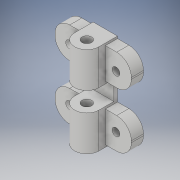
# Autodesk Inventor part: Nose Gear Mounting Block
Saved by Autodesk Inventor 2018 (Build 220112000, 112)
## iProperties
Created: 2018-08-04
Part Number: Nose Gear Mounting Block
Material: Generic
Document SubType Name: Modeling
Designer: Michael Gunderman
Density: 0.934608 g/cm^3
Appearance: Default
Mass: 5 g
Surface Area: 35.4129 cm^2
Volume: 5.34984 cm^3
Author: Michael Gunderman
Autodesk Inventor part; units mm, degrees
ref_plane "YZ Plane" through (0, 0, 0) normal (1, 0, 0) x (0, 1, 0)
ref_plane "XZ Plane" through (0, 0, 0) normal (0, 1, 0) x (-1, 0, 0)
ref_plane "XY Plane" through (0, 0, 0) normal (0, 0, 1) x (1, 0, 0)
sketch "Sketch1" plane through (0, 0, 0) normal (0, 0, 1) x (1, 0, 0)
  line L0 (0, 0) -> (10, 0)
  line L1 (10, 0) -> (10, 37.084)
  line L2 (10, 37.084) -> (0, 37.084)
  line L3 (0, 37.084) -> (0, 0)
  line L4 (0, 36.191) -> (-10.668, 36.191)
  line L5 (-10.668, 36.191) -> (-10.668, 23.491)
  line L6 (-10.668, 23.491) -> (0, 23.491)
  line L7 (0, 23.491) -> (0, 36.191)
  line L8 (0, 0.9264) -> (-10.668, 0.9264)
  line L9 (-10.668, 0.9264) -> (-10.668, 13.6264)
  line L10 (-10.668, 13.6264) -> (0, 13.6264)
  line L11 (0, 13.6264) -> (0, 0.9264)
  line L12 (5, 37.084) -> (5, 9.6109) construction
  line L13 (10, 36.191) -> (20.668, 36.191)
  line L14 (20.668, 36.191) -> (20.668, 23.491)
  line L15 (20.668, 23.491) -> (10, 23.491)
  line L16 (10, 0.9264) -> (20.668, 0.9264)
  line L17 (20.668, 0.9264) -> (20.668, 13.6264)
  line L18 (20.668, 13.6264) -> (10, 13.6264)
  line L19 (10, 36.191) -> (10, 23.491)
  line L20 (10, 13.6264) -> (10, 0.9264)
  dimension "d0" = 10
  dimension "d1" = 37.084
  dimension "d2" = 10.668
  dimension "d3" = 12.7
  dimension "d4" = 10.668
  dimension "d5" = 12.7
  constraints: 42 end point, 8 symmetric about line, 6 parallel, 5 perpendicular, 3 horizontal, 2 point on line, 1 midpoint, 1 vertical
  measures "d0" distance of L2.end L1.end
  measures "d1" distance of L1.end L0.end
  measures "d2" distance of L6.end L5.end
  measures "d3" distance of L5.end L4.end
  measures "d4" distance of L9.end L10.end
  measures "d5" distance of L8.end L9.end
extrude "Extrusion1" add sketch "Sketch1" along normal blind 12.61 contours L3 L2 L1 L0
extrude "Extrusion2" add sketch "Sketch1" along normal blind 5 contours L8 L9 L10 L3 | L6 L5 L4 L3
extrude "Extrusion3" add sketch "Sketch1" along normal blind 5 contours L1 L18 L17 L16 | L1 L13 L14 L15
fillet "Fillet1" radius 5 2 edges at (10, 18.542, 12.61) (0, 18.542, 12.61)
fillet "Fillet2" radius 6 8 edges at (20.668, 36.191, 2.5) (20.668, 23.491, 2.5) (20.668, 13.6264, 2.5) (20.668, 0.9264, 2.5) (-10.668, 13.6264, 2.5) (-10.668, 36.191, 2.5) (-10.668, 23.491, 2.5) (-10.668, 0.9264, 2.5)
sketch "Sketch2" plane through (0, 0, 5) normal (0, 0, 1) x (1, 0, 0)
  arc A0 (-4.668, 13.6264) -> (-10.668, 7.6264) centre (-4.668, 7.6264) ccw projected
  circle A1 centre (-4.668, 7.6264) radius 1.5875
  line L0 (-4.668, 7.6264) -> (-4.668, 29.2164) construction
  line L1 (-4.668, 29.2164) -> (14.382, 29.2164) construction
  circle A2 centre (-4.668, 29.2164) radius 1.5875
  circle A3 centre (14.382, 29.2164) radius 1.5875
  circle A4 centre (14.382, 7.6264) radius 1.5875
  point P0 (0, 0)
  dimension "d14" = 3.175
  dimension "d15" = 21.59
  dimension "d16" = 19.05
  dimension "d17" = 3.175
  dimension "d18" = 3.175
  dimension "d19" = 3.175
  constraints: 4 centre point, 4 end point, 3 coincident, 1 horizontal, 1 vertical
  measures "d14" diameter of A1
  measures "d15" distance of L0.start L0.end
  measures "d16" distance of L0.end L1.end
  measures "d17" diameter of A2
  measures "d18" diameter of A3
  measures "d19" diameter of A4
extrude "Extrusion4" cut sketch "Sketch2" against normal blind 5
sketch "Sketch3" plane through (0, 0, 0) normal (0, -1, 0) x (1, 0, 0)
  arc A0 (10, 7.61) -> (0, 7.61) centre (5, 7.61) ccw projected
  circle A1 centre (5, 7.61) radius 2
  point P0 (0, 0)
  dimension "d22" = 4
  constraints: 1 centre point, 1 coincident
  measures "d22" diameter of A1
extrude "Extrusion5" cut sketch "Sketch3" against normal blind 100
ref_plane "Work Plane1" through (0, 18.542, 0) normal (0, 1, 0) x (1, 0, 0)
sketch "Sketch4" plane through (0, 18.542, 0) normal (0, 1, 0) x (1, 0, 0)
  arc A0 (0, -7.61) -> (10, -7.61) centre (5, -7.61) ccw construction
  line L0 (5, -12.61) -> (5, -1.47) construction
  line L1 (10, -1.47) -> (0, -1.47)
  line L2 (0, 0) -> (0, -7.61) projected
  line L3 (0, -1.47) -> (-2.5969, -14.0453)
  line L4 (-2.5969, -14.0453) -> (12.3635, -14.2385)
  line L5 (12.3635, -14.2385) -> (10, -1.47)
  dimension "d25" = 11.14
  constraints: 10 end point, 1 horizontal, 1 point on circle, 1 point on line, 1 vertical
  measures "d25" distance of L0.start L0.end
extrude "Extrusion6" cut sketch "Sketch4" along normal mid plane 8
body "Solid1"
